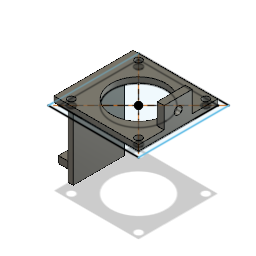
StórUppNiðurFesting v1 (Autodesk Fusion 360 design; units mm, degrees)
Autodesk Fusion 360 part; units mm, degrees
note: some values were not read from the file. Set by a fixed rule: which sketch regions a step uses.
sketch "Sketch1" plane through (0, 0, 0) normal (0, 1, 0) x (1, 0, 0)
  line L0 (28.15, 28.15) -> (-28.15, 28.15)
  line L1 (-28.15, 28.15) -> (-28.15, -28.15)
  line L2 (-28.15, -28.15) -> (28.15, -28.15)
  line L3 (28.15, -28.15) -> (28.15, 28.15)
  line L4 (28.15, 28.15) -> (-28.15, -28.15) construction
  line L5 (-28.15, 28.15) -> (28.15, -28.15) construction
  line L6 (28.15, 28.15) -> (23.85, 28.15)
  line L7 (23.85, 28.15) -> (23.85, 23.85)
  circle A0 centre (23.85, 23.85) radius 2.5
  circle A1 centre (-23.85, 23.85) radius 2.5
  circle A2 centre (-23.85, -23.85) radius 2.5
  circle A3 centre (23.85, -23.85) radius 2.5
  line L8 (32, 32) -> (-32, 32)
  line L9 (-32, 32) -> (-32, -32)
  line L10 (-32, -32) -> (32, -32)
  line L11 (32, -32) -> (32, 32)
  line L12 (32, 32) -> (-32, -32) construction
  line L13 (-32, 32) -> (32, -32) construction
  circle A4 centre (0, 0) radius 19.25
  dimension "d1" = 56.3
  dimension "d2" = 56.3
  dimension "d3" = 4.3
  dimension "d4" = 4.3
  dimension "d5" = 5
  dimension "d7" = 360
  dimension "d8" = 64
  dimension "d9" = 38.5
  constraint horizontal L0
  constraint perpendicular L0 L1
  constraint parallel L0 L2
  constraint parallel L1 L3
  constraint coincident L4 A4.centre
  constraint coincident L5 A4.centre
  constraint coincident A4.centre origin
  constraint perpendicular L3 L6
  constraint perpendicular L6 L7
  constraint coincident L7.end A0.centre
  constraint horizontal L8
  constraint perpendicular L8 L9
  constraint parallel L8 L10
  constraint parallel L9 L11
  constraint coincident L12 A4.centre
  constraint coincident L13 A4.centre
  measures "d1" distance of L1.end L2.end
  measures "d2" distance of L0.end L1.end
  measures "d3" distance of L0.start L6.end
  measures "d4" distance of L6.end L7.end
  measures "d5" diameter of A0
  measures "d8" distance of L8.end L9.end
  measures "d9" diameter of A4
extrude "Extrude1" add sketch "Sketch1" along normal blind 4 contours L0 L1 L2 L3 L6 | L8 L9 L10 L11
sketch "Sketch2" plane through (0, 0, 0) normal (0, 1, 0) x (1, 0, 0)
  circle A0 centre (-23.85, 23.85) radius 2.5
  circle A1 centre (23.85, 23.85) radius 2.5
  circle A2 centre (0, 0) radius 19.25
  circle A3 centre (23.85, -23.85) radius 2.5
  circle A4 centre (-23.85, -23.85) radius 2.5
  line L0 (32, 32) -> (32, -32)
  line L1 (32, -32) -> (-32, -32)
  line L2 (-32, -32) -> (-32, 32)
  line L3 (-32, 32) -> (32, 32)
  line L4 (-28.15, 28.15) -> (-28.15, -28.15)
  line L5 (-32, 32) -> (-32, -32)
  line L6 (-28.15, -28.15) -> (-32, -28.15)
  line L7 (-28.15, 28.15) -> (-32, 28.15)
  constraint coincident L4.end L6.start
  constraint coincident L2 L6.end
  constraint perpendicular L2 L6
  constraint coincident L4.start L7.start
  constraint coincident L5 L7.end
  constraint perpendicular L5 L7
extrude "Extrude2" add sketch "Sketch2" against normal blind 54.2 contours L2 L4 L5 L6 L7
sketch "Sketch3" plane through (-32, 0, 0) normal (-1, 0, 0) x (0, 0, 1)
  line L0 (-32, 0) -> (-28.15, 0)
  line L1 (-28.15, 0) -> (-28.15, -54.2)
  line L2 (-28.15, -54.2) -> (28.15, -54.2)
  line L3 (28.15, -54.2) -> (28.15, 0)
  line L4 (28.15, 0) -> (32, 0)
  line L5 (32, 0) -> (32, 4)
  line L6 (32, 4) -> (-32, 4)
  line L7 (-32, 4) -> (-32, 0)
  line L8 (0, -54.2) -> (10, -54.2)
  line L9 (10, -54.2) -> (-10, -54.2)
  line L10 (-10, -54.2) -> (-10, -49.2)
  line L11 (-10, -49.2) -> (10, -49.2)
  line L12 (10, -49.2) -> (10, -54.2)
  dimension "d14" = 10
  dimension "d15" = 20
  dimension "d16" = 5
  constraint midpoint L2 L8.start
  constraint parallel L2 L8
  constraint horizontal L9
  constraint vertical L10
  constraint horizontal L11
  constraint vertical L12
  measures "d14" distance of L8.start L8.end
  measures "d15" distance of L8.end L9.end
  measures "d16" distance of L8.end L11.end
extrude "Extrude3" add sketch "Sketch3" along normal blind 15 contours L2 L8 L9 L10 L11 L12
sketch "Sketch4" plane through (0, -49.2, 0) normal (0, 1, 0) x (-1, 0, 0)
  line L0 (32, 10) -> (32, -10)
  line L1 (32, -10) -> (47, -10)
  line L2 (47, -10) -> (47, 10)
  line L3 (47, 10) -> (32, 10)
  line L4 (32, 0) -> (39, 0)
  circle A0 centre (39, 0) radius 2.75
  dimension "d19" = 7
  dimension "d20" = 5.5
  constraint midpoint L0 L4.start
  constraint perpendicular L0 L4
  constraint coincident L4.end A0.centre
  measures "d19" distance of L4.start L4.end
  measures "d20" diameter of A0
extrude "Extrude4" cut sketch "Sketch4" against normal blind 19 contours A0
extrude "Extrude7" cut sketch "Sketch1" along normal blind 5 contours L8 L9 L10 L11
sketch "Sketch7" plane through (0, 0, 0) normal (0, 1, 0) x (1, 0, 0)
  line L0 (-28.15, 28.15) -> (-28.15, -28.15)
  line L1 (-28.15, -28.15) -> (28.15, -28.15)
  line L2 (28.15, -28.15) -> (28.15, 28.15)
  line L3 (28.15, 28.15) -> (-28.15, 28.15)
  circle A0 centre (-23.85, 23.85) radius 2.5
  circle A1 centre (23.85, 23.85) radius 2.5
  circle A2 centre (0, 0) radius 19.25
  circle A3 centre (23.85, -23.85) radius 2.5
  circle A4 centre (-23.85, -23.85) radius 2.5
  line L4 (-28.15, -28.15) -> (-32, -28.15)
  line L5 (-28.15, 28.15) -> (-32, 28.15)
  line L6 (-32, 28.15) -> (-32, -28.15)
  line L7 (-28.15, -28.15) -> (-28.15, 28.15)
  constraint coincident L0.end L1.start
  constraint perpendicular L0 L4
  constraint coincident L0.start L3.end
  constraint perpendicular L0 L5
  constraint perpendicular L4 L6
extrude "Extrude8" add sketch "Sketch7" along normal blind 4 contours L0 L4 L5 L6 L7
sketch "Sketch8" plane through (-28.15, 0, 0) normal (1, 0, 0) x (0, 0, -1)
  line L0 (28.15, 0) -> (-28.15, 0)
  line L1 (-28.15, 0) -> (-28.15, -54.2)
  line L2 (-28.15, -54.2) -> (28.15, -54.2)
  line L3 (28.15, -54.2) -> (28.15, 0)
  line L4 (-28.15, -54.2) -> (-18.15, -54.2)
  line L5 (-18.15, -54.2) -> (-28.15, -54.2)
  line L6 (-28.15, -54.2) -> (-28.15, 0)
  line L7 (-28.15, 0) -> (-18.15, 0)
  line L8 (-18.15, 0) -> (-18.15, -54.2)
  line L9 (28.15, -54.2) -> (18.15, -54.2)
  line L10 (18.15, -54.2) -> (28.15, -54.2)
  line L11 (28.15, -54.2) -> (28.15, 0)
  line L12 (28.15, 0) -> (18.15, 0)
  line L13 (18.15, 0) -> (18.15, -54.2)
  dimension "d36" = 10
  dimension "d37" = 10
  constraint coincident L1.end L2.start
  constraint perpendicular L1 L4
  constraint horizontal L5
  constraint vertical L6
  constraint horizontal L7
  constraint vertical L8
  constraint coincident L0.end L1.start
  constraint coincident L2.end L3.start
  constraint perpendicular L3 L9
  constraint horizontal L10
  constraint vertical L11
  constraint horizontal L12
  constraint vertical L13
  constraint coincident L0.start L3.end
  measures "d36" distance of L1.end L4.end
  measures "d37" distance of L2.end L9.end
extrude "Extrude9" cut sketch "Sketch8" against normal blind 4 contours L0 L2 L3 L9 L10 L11 L12 L13 | L0 L1 L2 L4 L5 L6 L7 L8
sketch "Sketch9" plane through (0, 4, 0) normal (0, 1, 0) x (-1, 0, 0)
  line L0 (32, 28.15) -> (-28.15, 28.15)
  line L1 (-28.15, 28.15) -> (-28.15, -28.15)
  line L2 (-28.15, -28.15) -> (32, -28.15)
  line L3 (32, -28.15) -> (32, 28.15)
  circle A0 centre (23.85, -23.85) radius 2.5
  circle A1 centre (-23.85, -23.85) radius 2.5
  circle A2 centre (0, 0) radius 19.25
  circle A3 centre (-23.85, 23.85) radius 2.5
  circle A4 centre (23.85, 23.85) radius 2.5
  line L4 (-28.15, 0) -> (-28.15, -10)
  line L5 (-28.15, -10) -> (-23.15, -10)
  line L6 (-23.15, -10) -> (-23.15, 10)
  line L7 (-23.15, 10) -> (-28.15, 10)
  line L8 (-28.15, 10) -> (-28.15, -10)
  dimension "d40" = 10
  dimension "d41" = 5
  dimension "d42" = 20
  constraint midpoint L1 L4.start
  constraint parallel L1 L4
  constraint horizontal L5
  constraint vertical L6
  constraint horizontal L7
  constraint vertical L8
  measures "d40" distance of L4.start L4.end
  measures "d41" distance of L4.end L5.end
  measures "d42" distance of L4.end L7.end
extrude "Extrude10" add sketch "Sketch9" along normal blind 15 contours L1 L4 L5 L6 L7 L8
sketch "Sketch10" plane through (23.15, 0, 0) normal (-1, 0, 0) x (0, 0, 1)
  line L0 (-10, 4) -> (10, 4)
  line L1 (10, 4) -> (10, 19)
  line L2 (10, 19) -> (-10, 19)
  line L3 (-10, 19) -> (-10, 4)
  line L4 (0, 4) -> (0, 11)
  circle A0 centre (0, 11) radius 2.8
  dimension "d45" = 7
  dimension "d46" = 5.6
  constraint midpoint L0 L4.start
  constraint perpendicular L0 L4
  constraint coincident L4.end A0.centre
  measures "d45" distance of L4.start L4.end
  measures "d46" diameter of A0
extrude "Extrude11" cut sketch "Sketch10" against normal blind 13 contours A0
